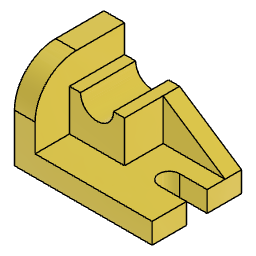
Design 6 v1 (Autodesk Fusion 360 design; units mm, degrees)
Autodesk Fusion 360 part; units mm, degrees
box "BoxPrimitive1" add length 650 width 1000 height 150 placed x (0, -1, 0) y (1, 0, 0) z (0, 0, 1) at (0, 0, 0)
sketch "Sketch3" plane through (0, 0, 150) normal (0, 0, 1) x (-1, 0, 0)
  line L0 (0, 650) -> (-1000, 650)
  line L1 (-1000, 650) -> (-1000, 0)
  line L2 (-1000, 0) -> (0, 0)
  line L3 (0, 0) -> (0, 650)
  line L4 (0, 0) -> (-150, 0)
  line L5 (-150, 0) -> (-150, 650)
  line L6 (-150, 650) -> (0, 650)
  line L7 (0, 650) -> (0, 0)
  line L8 (-150, 0) -> (-550, 0)
  line L9 (-550, 0) -> (-550, 400)
  line L10 (-550, 400) -> (-150, 400)
  line L11 (-150, 400) -> (-150, 0)
  line L12 (-550, 0) -> (-1000, 0)
  line L13 (-1000, 0) -> (-1000, 120)
  line L14 (-1000, 120) -> (-550, 120)
  line L15 (-550, 120) -> (-550, 0)
  line L16 (-800, 250) -> (-1000, 250)
  line L17 (-1000, 250) -> (-1000, 400)
  line L18 (-1000, 400) -> (-800, 400)
  arc A0 (-800, 250) -> (-800, 400) centre (-800, 325) ccw
  dimension "d6" = 150
  dimension "d7" = 400
  dimension "d8" = 400
  dimension "d9" = 120
  dimension "d10" = 150
  dimension "d11" = 200
  constraint horizontal L4
  constraint vertical L5
  constraint horizontal L6
  constraint vertical L7
  constraint coincident L0 L5.end
  constraint coincident L2.end L3.start
  constraint horizontal L8
  constraint vertical L9
  constraint horizontal L10
  constraint vertical L11
  constraint horizontal L12
  constraint vertical L13
  constraint horizontal L14
  constraint vertical L15
  constraint horizontal L16
  constraint vertical L17
  constraint horizontal L18
  constraint coincident L1 L17.end
  measures "d6" distance of L2.end L4.end
  measures "d7" distance of L4.end L8.end
  measures "d8" distance of L4.end L10.end
  measures "d9" distance of L8.end L14.end
  measures "d10" diameter of A0
  measures "d11" distance of L1 A0.centre
extrude "Extrude1" add sketch "Sketch3" along normal blind 500 contours L0 L2 L3 L4 L5 L6 L7 L11
extrude "Extrude2" add sketch "Sketch3" along normal blind 300 contours L2 L5 L8 L9 L10 L11 L15 | L1 L2 L9 L12 L13 L14 L15
extrude "Extrude3" cut sketch "Sketch3" against normal blind 300 contours L1 L16 L17 L18 A0
fillet "Fillet1" radius 300 1 edges at (75, -650, 650)
chamfer "Chamfer1" distance 450 distance2 300 1 edges at (1000, -60, 450) measured on face at (283.3333, -173.3333, 450)
sketch "Sketch4" plane through (0, 0, 450) normal (0, 0, 1) x (-1, 0, 0)
  line L0 (-550, 120) -> (-550, 0)
  line L1 (-550, 0) -> (-150, 0)
  line L2 (-150, 0) -> (-150, 400)
  line L3 (-150, 400) -> (-550, 400)
  line L4 (-550, 400) -> (-550, 120)
  line L5 (-350, 0) -> (-470, 0)
  line L6 (-470, 0) -> (-470, 400)
  line L7 (-470, 400) -> (-350, 400)
  line L8 (-350, 400) -> (-350, 0)
  dimension "d22" = 120
  dimension "d23" = 400
  constraint horizontal L5
  constraint vertical L6
  constraint horizontal L7
  constraint vertical L8
  constraint midpoint L1 L5.start
  measures "d22" distance of L5.start L5.end
  measures "d23" distance of L5.start L7.end
revolve "Revolve1" cut sketch "Sketch4" angle 360 about axis through (350, -400, 450) along (0, 1, 0) contours L1 L3 L5 L6 L7 L8
